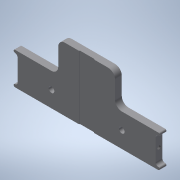
# Autodesk Inventor part: Grundplatte
Saved by Autodesk Inventor 2022 (Build 260153000, 153)
## iProperties
Created: 2014-03-25
Part Number: Grundplatte
Material: Generisch
Document SubType Name: Modeling
Designer: g.schardt
Density: 1 g/cm^3
Appearance: Vorgabe
Project: 10W LED Tauchlampe
Author: schardt
Autodesk Inventor part; units mm, degrees
ref_plane "YZ Plane" through (0, 0, 0) normal (1, 0, 0) x (0, 1, 0)
ref_plane "XZ Plane" through (0, 0, 0) normal (0, 1, 0) x (-1, 0, 0)
sketch "Skizze1" plane through (0, 0, 0) normal (0, 1, 0) x (-1, 0, 0)
  line L0 (-54, 0) -> (54, 0)
  line L1 (54, 0) -> (54, 24)
  line L2 (54, 24) -> (21, 24)
  line L3 (21, 24) -> (21, 47)
  line L4 (21, 47) -> (-21, 47)
  line L5 (-21, 47) -> (-21, 24)
  line L6 (-21, 24) -> (-54, 24)
  line L7 (-54, 24) -> (-54, 0)
  point P0 (0, 0)
  point P1 (0, 0)
  dimension "d0" = 108
  dimension "d1" = 24
  dimension "d2" = 33
  dimension "d3" = 23
  dimension "d4" = 42
  constraints: 16 end point, 3 parallel, 3 perpendicular, 2 collinear, 1 coincident, 1 horizontal, 1 midpoint
  measures "d0" distance of L0.start L0.end
  measures "d1" distance of L0.end L1.end
  measures "d2" distance of L1.end L2.end
  measures "d3" distance of L2.end L3.end
  measures "d4" distance of L3.end L4.end
extrude "Extrusion1" add sketch "Skizze1" along normal blind 5
sketch "Skizze2" plane through (54, 0, 24) normal (1, 0, 0) x (0, 0, -1)
  line L0 (0, 0) -> (24, 0) projected
  line L1 (24, 0) -> (24, 5) projected
  line L2 (0, 5) -> (24, 5) projected
  line L3 (0, 0) -> (0, 5) projected
  line L4 (2, 0) -> (22, 0)
  line L5 (22, 0) -> (22, 5)
  line L6 (22, 5) -> (2, 5)
  line L7 (2, 5) -> (2, 0)
  dimension "d7" = 2
  dimension "d8" = 2
  constraints: 8 end point, 2 parallel, 2 point on line, 1 horizontal, 1 perpendicular
  measures "d7" distance between parallel lines of L3 L7
  measures "d8" distance between parallel lines of L1 L5
extrude "Extrusion2" cut sketch "Skizze2" against normal blind 3 contours L7 L2 L5 L0
sketch "Skizze3" plane through (-54, 0, 0) normal (-1, 0, 0) x (0, 0, 1)
  line L0 (0, 0) -> (24, 0) projected
  line L1 (24, 0) -> (24, 5) projected
  line L2 (0, 5) -> (24, 5) projected
  line L3 (0, 0) -> (0, 5) projected
  line L4 (2, 0) -> (22, 0)
  line L5 (22, 0) -> (22, 5)
  line L6 (22, 5) -> (2, 5)
  line L7 (2, 5) -> (2, 0)
  dimension "d11" = 2
  dimension "d12" = 2
  constraints: 8 end point, 2 parallel, 2 point on line, 1 horizontal, 1 perpendicular
  measures "d11" distance between parallel lines of L3 L7
  measures "d12" distance between parallel lines of L1 L5
extrude "Extrusion3" cut sketch "Skizze3" against normal blind 3 contours L7 L2 L5 L0
fillet "Rundung1" radius 1 8 edges at (-54, 2.5, 0) (-54, 2.5, 2) (-54, 2.5, 22) (-54, 2.5, 24) (54, 2.5, 24) (54, 2.5, 22) (54, 2.5, 2) (54, 2.5, 0)
fillet "Rundung2" radius 5 4 edges at (21, 2.5, 24) (21, 2.5, 47) (-21, 2.5, 47) (-21, 2.5, 24)
sketch "Skizze4" plane through (53, 0, 0) normal (0, 0, -1) x (-1, 0, 0)
  line L0 (58.5, -0.5) -> (47.5, -0.5)
  line L1 (47.5, -0.5) -> (47.5, 0.5)
  line L2 (47.5, 0.5) -> (58.5, 0.5)
  line L3 (58.5, 0.5) -> (58.5, -0.5)
  line L4 (58.5, -0.5) -> (47.5, 0.5) construction
  line L5 (47.5, -0.5) -> (58.5, 0.5) construction
  point P0 (53, 0)
  dimension "d17" = 11
  dimension "d18" = 1
  constraints: 12 end point, 2 midpoint, 2 parallel, 1 horizontal, 1 perpendicular
  measures "d17" distance of L1.end L2.end
  measures "d18" distance of L0.end L1.end
extrude "Extrusion4" cut sketch "Skizze4" against normal through all
sketch "Skizze6" plane through (0, 5, 0) normal (0, 1, 0) x (1, 0, 0)
  line L0 (53, 0) -> (-53, 0) projected
  point P0 (0, 0)
  point P1 (-26, -12)
  point P2 (26, -12)
  dimension "d31" = 12
  dimension "d32" = 26
  dimension "d33" = 26
  constraints: 1 horizontal alignment
  measures "d31" distance from line of L0 point (-26, -12)
  measures "d32" horizontal distance of point (0, 0) point (-26, -12)
  measures "d33" horizontal distance of point (0, 0) point (26, -12)
hole "Bohrung2" at (-26, 5, 12) at (26, 5, 12) direction (0, -1, 0) diameter 4.2 end through all countersink diameter 8.4 countersink angle 90
sketch "Skizze7" plane through (51, 0, 24) normal (1, 0, 0) x (0, 0, -1)
  line L0 (22, 5) -> (22, 0) projected
  line L1 (2, 5) -> (22, 5) projected
  point P0 (24, 0)
  point P1 (12, 2.5)
  dimension "d41" = 2.5
  dimension "d42" = 10
  measures "d41" distance from line of L1 point (12, 2.5)
  measures "d42" distance from line of L0 point (12, 2.5)
hole "Bohrung3" at (51, 2.5, 12) direction (-1, 0, 0) diameter 2.459 depth 6 tip angle 118 thread size "M3x0.5" class "6H" standard "ANSI Metric M Profile"
sketch "Skizze8" plane through (-51, 0, 0) normal (-1, 0, 0) x (0, 0, 1)
  line L0 (2, 5) -> (22, 5) projected
  line L1 (2, 0) -> (2, 5) projected
  point P0 (0, 0)
  point P1 (12, 2.5)
  dimension "d50" = 2.5
  dimension "d51" = 10
  measures "d50" distance from line of L0 point (12, 2.5)
  measures "d51" distance from line of L1 point (12, 2.5)
hole "Bohrung4" at (-51, 2.5, 12) direction (1, 0, 0) diameter 2.459 depth 6 tip angle 118 thread size "M3x0.5" class "6H" standard "ANSI Metric M Profile"
ref_plane "Arbeitsebene1" through (-51, 0, 12) normal (0, 0, -1) x (-1, 0, 0)
fillet "Rundung3" radius 2 2 edges at (51, 2.5, 2) (51, 2.5, 22)
fillet "Rundung4" radius 2 2 edges at (-51, 2.5, 22) (-51, 2.5, 2)
